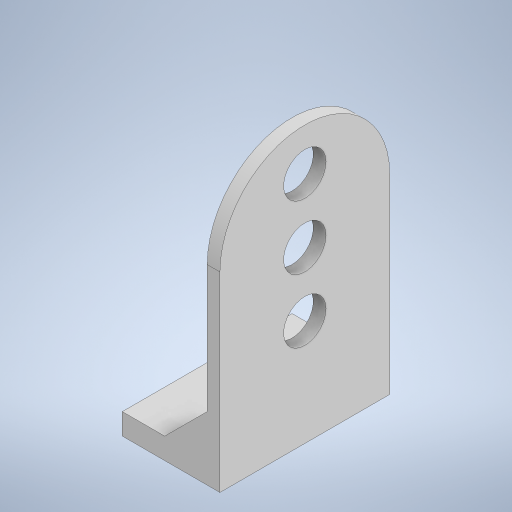
# Autodesk Inventor part: pot_stand
Saved by Autodesk Inventor 2023 (Build 270158000, 158)
## iProperties
Created: 2022-11-10
Part Number: pot_stand
Material: Generic
Document SubType Name: Modeling
Designer: eahil
Density: 1 g/cm^3
Appearance: Default
Author: eahil
Autodesk Inventor part; units mm, degrees
ref_plane "YZ Plane" through (0, 0, 0) normal (1, 0, 0) x (0, 1, 0)
ref_plane "XZ Plane" through (0, 0, 0) normal (0, 1, 0) x (-1, 0, 0)
ref_plane "XY Plane" through (0, 0, 0) normal (0, 0, 1) x (1, 0, 0)
sketch "Sketch1" plane through (0, 0, 0) normal (1, 0, 0) x (0, 1, 0)
  line L0 (0, 0) -> (65, 0)
  line L1 (65, 0) -> (65, -40)
  line L2 (65, -40) -> (0, -40)
  line L3 (0, -40) -> (0, 0)
  dimension "d0" = 40
  dimension "d1" = 65
  constraints: 8 end point, 2 parallel, 1 horizontal, 1 perpendicular
  measures "d0" distance of L2.end L0.start
  measures "d1" distance of L1.end L2.end
extrude "Extrusion1" add sketch "Sketch1" along normal blind 3
sketch "Sketch2" plane through (0, 0, 0) normal (-1, 0, 0) x (0, 0, 1)
  line L0 (0, 0) -> (-40, 0) projected
  line L1 (-40, 0) -> (-40, 65) projected
  line L2 (0, 0) -> (-40, 0)
  line L3 (-40, 0) -> (-40, 5)
  line L4 (-40, 5) -> (0, 5)
  line L5 (0, 5) -> (0, 0)
  dimension "d4" = 5
  constraints: 8 end point, 2 parallel, 1 horizontal, 1 perpendicular, 1 point on line
  measures "d4" distance between parallel lines of L0 L4
extrude "Extrusion2" add sketch "Sketch2" along normal blind 20
chamfer "Chamfer1" distance 10 angle 45 1 edges at (0, 5, -20)
sketch "Sketch3" plane through (3, 0, 0) normal (1, 0, 0) x (0, 0, -1)
  circle A0 centre (20, 55) radius 5
  circle A1 centre (20, 40) radius 5
  circle A2 centre (20, 25) radius 5
  line L0 (40, 65) -> (0, 65) projected
  point P0 (0, 0)
  dimension "d10" = 10
  dimension "d11" = 10
  dimension "d12" = 5
  dimension "d13" = 15
  dimension "d14" = 20
  constraints: 3 centre point, 2 equal radius, 2 vertical alignment
  measures "d10" diameter of A0
  measures "d11" distance from line of L0 A0.centre
  measures "d13" distance of A2.centre A1.centre
  measures "d14" horizontal distance of L0.start A0.centre
extrude "Extrusion3" cut sketch "Sketch3" against normal up to surface (3 mm away)
fillet "Fillet1" radius 20 2 edges at (1.5, 65, 0) (1.5, 65, -40)
body "Solid1"
